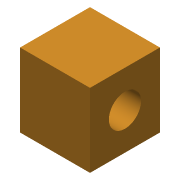
# Autodesk Inventor part: 3136 1094 44
Saved by Autodesk Inventor 2022 Beta2 (Build 260130000, 130) ContinuousBuild 0
## iProperties
Shininess: 64.0
Length Units: 11269
Angle Units: 11279
Time Units: 11290
Mass Units: 11283
Length Display Precision: 3
Angle Display Precision: 2
Compacted: True
Part Number: 3136 1094 44
Document SubType Name: Modeling
Created: 2003-04-13
Designer: Uffe Bak
Material: Steel, Mild
Density: 7.86 g/cm^3
Appearance: Brokk-Gul
Density: 0.0
Volumn: 0.0
Area: 0.0
PropertySet Name: Model Information
Control State: 0
Master: False
Checked Out: False
Author: Uffe Bak
Autodesk Inventor part; units mm, degrees
ref_plane "YZ Plane" through (0, 0, 0) normal (1, 0, 0) x (0, 1, 0)
ref_plane "XZ Plane" through (0, 0, 0) normal (0, 1, 0) x (-1, 0, 0)
ref_plane "XY Plane" through (0, 0, 0) normal (0, 0, 1) x (1, 0, 0)
sketch "Sketch1" plane through (0, 0, 0) normal (0, 0, 1) x (1, 0, 0)
  line L0 (38, 38) -> (38, -38)
  line L1 (38, -38) -> (-38, -38)
  line L2 (-38, -38) -> (-38, 38)
  line L3 (-38, 38) -> (38, 38)
  point P0 (0, 0)
  point P1 (0, 0)
  dimension "d0" = 76
  constraints: 8 end point, 1 coincident, 7 other
  measures "d0" distance of L2.end L0.start
extrude "Extrusion1" add sketch "Sketch1" along normal blind 80
sketch "Sketch2" plane through (38, -38, 0) normal (1, 0, 0) x (0, 0, -1)
  line L0 (0, 76) -> (0, 0) projected
  circle A0 centre (-40, 38) radius 17.5
  line L1 (0, 38) -> (-40, 38) construction
  dimension "d3" = 40
  dimension "d4" = 35
  constraints: 2 end point, 1 centre point, 1 horizontal, 1 midpoint
  measures "d3" distance from line of L0 L1.end
  measures "d4" diameter of A0
extrude "Extrusion2" cut sketch "Sketch2" against normal through all
body "Solid1"
